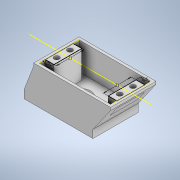
# Autodesk Inventor part: Übersetzungsbox_2
Saved by Autodesk Inventor 2021 (Build 250183000, 183)
## iProperties
Created: 2021-01-10
Part Number: Übersetzungsbox_2
Material: Generisch
Document SubType Name: Modeling
Designer: Ctroi
Density: 1 g/cm^3
Appearance: Vorgabe
Author: Ctroi
## iProperties of the stored document _3D-Druck.ipt
Created: 2021-01-13
Part Number: _3D-Druck
Material: Generisch
Document SubType Name: Modeling
Designer: Ctroi
Density: 1 g/cm^3
Appearance: Vorgabe
Author: Ctroi
Autodesk Inventor part; units mm, degrees
ref_plane "YZ Plane" through (0, 0, 0) normal (1, 0, 0) x (0, 1, 0)
ref_plane "XZ Plane" through (0, 0, 0) normal (0, 1, 0) x (-1, 0, 0)
ref_plane "XY Plane" through (0, 0, 0) normal (0, 0, 1) x (1, 0, 0)
sketch "Skizze1" plane through (0, 0, 0) normal (0, 1, 0) x (-1, 0, 0)
  line L0 (-26, -17.1) -> (26, -17.1)
  line L1 (26, -17.1) -> (26, 17.1)
  line L2 (26, 17.1) -> (-26, 17.1)
  line L3 (-26, 17.1) -> (-26, -17.1)
  line L4 (0, -23.94) -> (0, 23.94) projected
  line L5 (-36.4, 0) -> (36.4, 0) projected
  point P0 (0, 0)
  dimension "d0" = 52
  dimension "d1" = 34.2
  constraints: 8 end point, 2 parallel, 1 horizontal, 1 perpendicular, 2 other
  measures "d0" distance of L1.end L2.end
  measures "d1" distance of L0.end L1.end
extrude "Extrusion1" add sketch "Skizze1" along normal blind 6
ref_plane "Arbeitsebene1" through (0, 25, 0) normal (0, 1, 0) x (1, 0, 0)
sketch "Skizze2" plane through (0, 25, 0) normal (0, 1, 0) x (1, 0, 0)
  line L0 (26, 17.1) -> (-26, 17.1) projected
  line L1 (-18.7, 17.1) -> (39.3, 17.1)
  line L2 (39.3, 17.1) -> (39.3, -17.1)
  line L3 (39.3, -17.1) -> (-18.7, -17.1)
  line L4 (-18.7, -17.1) -> (-18.7, 17.1)
  line L5 (-26, 17.1) -> (-26, -17.1) projected
  point P0 (0, 0)
  dimension "d5" = 58
  dimension "d6" = 34.2
  dimension "d7" = 7.3
  constraints: 8 end point, 2 parallel, 1 horizontal, 1 perpendicular, 1 point on line
  measures "d5" distance of L2.end L3.end
  measures "d6" distance of L1.end L2.end
  measures "d7" distance between parallel lines of L5 L4
extrude "Extrusion2" add sketch "Skizze2" along normal blind 2
loft "Erhebung1" add section 1 edges at (-26, 6, 0) (0, 6, 17.1) (26, 6, 0) (0, 6, -17.1) section 2 edges at (39.3, 25, 0) (10.3, 25, 17.1) (-18.7, 25, 0) (10.3, 25, -17.1)
shell "Wandung1" thickness 2 removed faces 1 at (0.6333, 27, -5.7)
sketch "Skizze7" plane through (-24, 2, 15.1) normal (0, 1, 0) x (1, 0, 0)
  line L0 (-2, 32.2) -> (-2, -2) projected
  line L1 (50, 32.2) -> (-2, 32.2) projected
  line L2 (-2, -2) -> (50, -2)
  line L3 (50, -2) -> (50, 32.2)
  line L4 (50, 32.2) -> (-2, 32.2)
  line L5 (-2, 32.2) -> (-2, -2)
  line L6 (48, 0) -> (0, 0)
  line L7 (0, 0) -> (0, 30.2)
  line L8 (0, 30.2) -> (48, 30.2)
  line L9 (48, 30.2) -> (48, 0)
  point P0 (24, 15.1)
  dimension "d28" = 2
  constraints: 16 end point, 4 parallel, 2 perpendicular, 1 horizontal, 3 other
  measures "d28" distance between parallel lines of L2 L6
extrude "Extrusion5" add sketch "Skizze7" along normal blind 4 contours L6 L7 L8 L9
sketch "Skizze8" plane through (-24, 6, 15.1) normal (0, 1, 0) x (1, 0, 0)
  circle A0 centre (24, 15.1) radius 7.25
  line L0 (-2, 32.2) -> (-2, -2) projected
  line L1 (50, 32.2) -> (-2, 32.2) projected
  point P0 (24, 15.1)
  dimension "d31" = 14.5
  dimension "d32" = 26
  dimension "d33" = 17.1
  constraints: 1 centre point
  measures "d31" diameter of A0
  measures "d32" distance from line of L0 A0.centre
  measures "d33" distance from line of L1 A0.centre
extrude "Extrusion7" cut sketch "Skizze8" against normal blind 4
sketch "Skizze9" plane through (0, 2, 0) normal (0, 1, 0) x (1, 0, 0)
  circle A0 centre (0, 0) radius 5.25
  point P0 (0, 0)
  dimension "d38" = 10.5
  constraints: 1 centre point
  measures "d38" diameter of A0
extrude "Extrusion8" cut sketch "Skizze9" against normal up to surface (2 mm away)
sketch "Skizze11" plane through (0, 27, 0) normal (0, 1, 0) x (1, 0, 0)
  line L0 (-16.7, -15.1) -> (-16.7, 15.1) projected
  line L1 (-16.7, 10.5) -> (-10.2, 10.5)
  line L2 (-10.2, 10.5) -> (-10.2, -10.5)
  line L3 (-10.2, -10.5) -> (-16.7, -10.5)
  line L4 (-16.7, -10.5) -> (-16.7, 10.5)
  line L5 (52.36, 0) -> (-39.06, 0) projected
  line L6 (37.3, -15.1) -> (37.3, 15.1) projected
  line L7 (37.3, -10.5) -> (30.8, -10.5)
  line L8 (30.8, -10.5) -> (30.8, 10.5)
  line L9 (30.8, 10.5) -> (37.3, 10.5)
  line L10 (37.3, 10.5) -> (37.3, -10.5)
  point P0 (0, 0)
  dimension "d49" = 6.5
  dimension "d50" = 21
  dimension "d58" = 6.5
  dimension "d59" = 21
  constraints: 16 end point, 4 parallel, 2 horizontal, 2 perpendicular, 2 point on line, 2 other
  measures "d49" distance of L2.end L3.end
  measures "d50" distance of L1.end L2.end
  measures "d58" distance of L8.end L9.end
  measures "d59" distance of L7.end L8.end
extrude "Extrusion9" add sketch "Skizze11" against normal blind 6 contours L0 L5 L2 L3 | L0 L1 L2 L5
thicken "Verdickung1" operation add thickness 1 both sides no extend neighbours yes toward (-1, 0, 0) faces at (-16.7, 23.4193, -3.5) (-21.4716, 12.2097, 3.5)
extrude "Extrusion11" add sketch "Skizze11" against normal blind 12 contours L6 L7 L8 L5 | L5 L8 L9 L6
chamfer "Fase1" distance 7.1407 angle 35 1 edges at (37.3, 15, 0) measured on face at (37.3, 15.5, 0)
sketch "Skizze13" plane through (0, 27, 0) normal (0, 1, 0) x (1, 0, 0)
  circle A0 centre (-13.45, 5) radius 1.95
  line L0 (-10.2, -10.5) -> (-10.2, 10.5) projected
  circle A1 centre (-13.45, -5) radius 1.95
  line L1 (52.36, 0) -> (-39.06, 0) projected
  circle A2 centre (34.05, 5) radius 1.95
  line L2 (30.8, 10.5) -> (30.8, -10.5) projected
  circle A3 centre (34.05, -5) radius 1.95
  point P0 (0, 0)
  dimension "d65" = 3.9
  dimension "d66" = 3.25
  dimension "d67" = 3.9
  dimension "d68" = 5
  dimension "d69" = 5
  dimension "d70" = 3.25
  dimension "d71" = 3.9
  dimension "d72" = 3.25
  dimension "d73" = 5
  dimension "d74" = 3.9
  dimension "d75" = 3.25
  dimension "d76" = 5
  constraints: 4 centre point
  measures "d65" diameter of A0
  measures "d66" distance from line of L0 A0.centre
  measures "d67" diameter of A1
  measures "d68" distance from line of L1 A0.centre
  measures "d69" distance from line of L1 A1.centre
  measures "d70" distance from line of L0 A1.centre
  measures "d71" diameter of A2
  measures "d72" distance from line of L2 A2.centre
  measures "d73" distance from line of L1 A2.centre
  measures "d74" diameter of A3
  measures "d75" distance from line of L2 A3.centre
  measures "d76" distance from line of L1 A3.centre
extrude "Extrusion12" cut sketch "Skizze13" against normal blind 5.7
sketch "Skizze14" plane through (0, 21, 0) normal (0, -1, 0) x (1, 0, 0)
  line L0 (-10.2, 10.5) -> (-10.2, -10.5) projected
  line L1 (-17.023, -10.5) -> (-16.7, -10.5) projected
  line L2 (-10.2, 10.5) -> (-16.7, 10.5)
  line L3 (-16.7, 10.5) -> (-16.7, -10.5)
  line L4 (-16.7, -10.5) -> (-10.2, -10.5)
  line L5 (-10.2, -10.5) -> (-10.2, 10.5)
  point P0 (0, 0)
  constraints: 8 end point, 2 parallel, 1 horizontal, 1 perpendicular
extrude "Extrusion13" add sketch "Skizze14" along normal up to surface (15 mm away)
